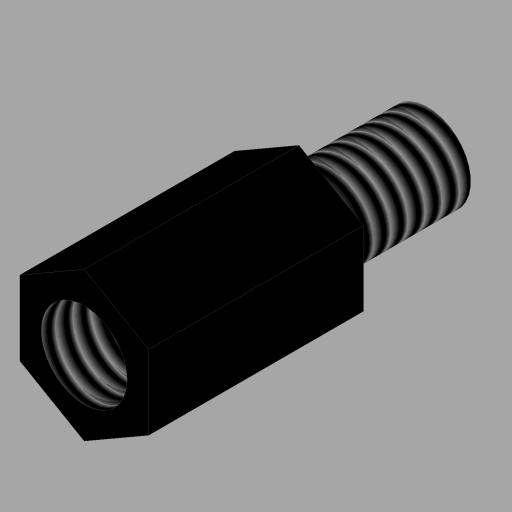
# Autodesk Inventor part: M2_5mm_standoff
Saved by Autodesk Inventor 2024 (Build 280153000, 153)
## iProperties
Created: 2024-02-14
Part Number: M2_5mm_standoff
Material: Generic
Document SubType Name: Modeling
Designer: critt
Density: 1 g/cm^3
Appearance: Default
Author: critt
Autodesk Inventor part; units mm, degrees
ref_plane "YZ Plane" through (0, 0, 0) normal (1, 0, 0) x (0, 1, 0)
ref_plane "XZ Plane" through (0, 0, 0) normal (0, 1, 0) x (-1, 0, 0)
ref_plane "XY Plane" through (0, 0, 0) normal (0, 0, 1) x (1, 0, 0)
sketch "Sketch1" plane through (0, 0, 0) normal (0, 0, 1) x (1, 0, 0)
  line L0 (0, 1.7321) -> (1.5, 0.866)
  line L1 (1.5, 0.866) -> (1.5, -0.866)
  line L2 (1.5, -0.866) -> (0, -1.7321)
  line L3 (0, -1.7321) -> (-1.5, -0.866)
  line L4 (-1.5, -0.866) -> (-1.5, 0.866)
  line L5 (-1.5, 0.866) -> (0, 1.7321)
  point P0 (0, 0)
  point P1 (0, 0)
  dimension "d0" = 3
  constraints: 12 end point, 1 coincident, 1 vertical, 13 other
  measures "d0" distance between parallel lines of L4 L1
extrude "Extrusion1" add sketch "Sketch1" along normal blind 5
sketch "Sketch2" plane through (0, 0, 5) normal (0, 0, 1) x (1, 0, 0)
  circle A0 centre (0, 0) radius 1
  dimension "d3" = 2
  constraints: 1 centre point, 1 coincident
  measures "d3" diameter of A0
extrude "Extrusion2" cut sketch "Sketch2" against normal blind 3
sketch "Sketch3" plane through (0, 0, 0) normal (0, 0, -1) x (-1, 0, 0)
  circle A0 centre (0, 0) radius 1
  constraints: 1 centre point, 1 coincident
extrude "Extrusion3" add sketch "Sketch3" along normal blind 3
thread "Thread1" size "M2x0.4" class "6g" standard "ANSI Metric M Profile" length 12.7
thread "Thread2" size "M2x0.4" class "6H" standard "ANSI Metric M Profile" length 12.7
body "Solid1"
